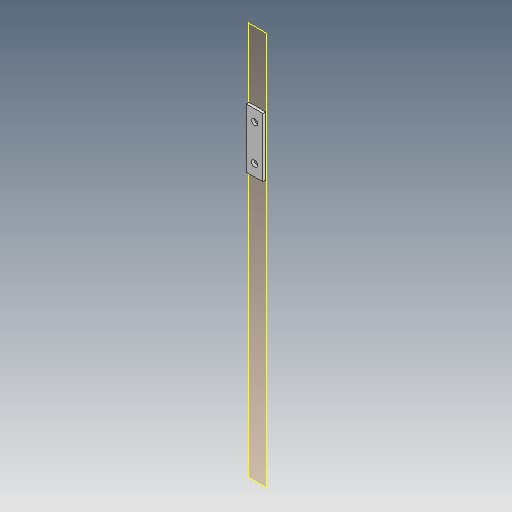
# Autodesk Inventor part: standoff for gripper servo
Saved by Autodesk Inventor 2020 (Build 240168000, 168)
## iProperties
Created: 2019-12-31
Part Number: standoff for gripper servo
Material: Generic
Document SubType Name: Modeling
Designer: ball
Density: 1 g/cm^3
Appearance: Default
Author: ball
Autodesk Inventor part; units mm, degrees
ref_plane "YZ Plane" through (0, 0, 0) normal (1, 0, 0) x (0, 1, 0)
ref_plane "XZ Plane" through (0, 0, 0) normal (0, 1, 0) x (-1, 0, 0)
ref_plane "XY Plane" through (0, 0, 0) normal (0, 0, 1) x (1, 0, 0)
ref_plane "Work Plane1" through (0, -0.0041, 0) normal (0, 0, 1) x (1, 0, 0)
sketch "Sketch1" plane through (0, -0.0041, 0) normal (0, 0, 1) x (1, 0, 0)
  line L0 (0, -194.9959) -> (0, 0.0041) construction
  line L1 (9, 0.0041) -> (9, -194.9959) construction
  circle A0 centre (4.5, -53.479) radius 1.7 construction
  circle A1 centre (4.5, -33.921) radius 1.7 construction
  circle A2 centre (4.5, -53.479) radius 1.7
  circle A3 centre (4.5, -33.921) radius 1.7
  line L2 (4.5, -53.479) -> (4.5, -59.829) construction
  line L3 (4.5, -33.921) -> (4.5, -27.571) construction
  line L4 (9, -27.5751) -> (0, -27.5751)
  line L5 (4.5, -59.829) -> (9, -59.829)
  line L6 (9, -27.5751) -> (9, -59.829)
  line L7 (4.5, -59.829) -> (0, -59.829)
  line L8 (0, -27.5751) -> (0, -59.829)
  dimension "d0" = 6.35
  dimension "d1" = 6.35
  constraints: 14 end point, 5 point on line, 2 centre point, 2 coincident, 2 concentric, 2 perpendicular, 2 vertical, 1 collinear, 1 horizontal
  measures "d0" distance of L2.start L2.end
  measures "d1" distance of L3.start L3.end
extrude "Extrusion1" add sketch "Sketch1" along normal blind 1.524
body "Solid1"
